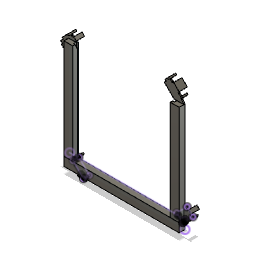
ClipOn v35 (Autodesk Fusion 360 design; units mm, degrees)
Autodesk Fusion 360 part; units mm, degrees
(part 1 of 2)
sketch "Sketch1" plane through (0, 0, 0) normal (0, 0, 1) x (1, 0, 0) in component "Faceplate"
  line L0 (10, 10) -> (310, 10)
  line L1 (310, 10) -> (310, 360)
  line L2 (310, 360) -> (10, 360)
  line L3 (10, 360) -> (10, 10)
  line L4 (85, 300) -> (235, 300)
  line L5 (235, 300) -> (235, 150)
  line L6 (235, 150) -> (85, 150)
  line L7 (85, 150) -> (85, 300)
  dimension "d7" = 10
  dimension "d8" = 10
  dimension "d10" = 350
  dimension "d11" = 75
  dimension "d12" = 140
  dimension "d13" = 150
  dimension "d14" = 150
  dimension "d15" = 75
  constraint horizontal L0
  constraint vertical L1
  constraint horizontal L2
  constraint vertical L3
  constraint horizontal L4
  constraint vertical L5
  constraint horizontal L6
  constraint vertical L7
  measures "d7" horizontal distance of origin L0.start
  measures "d8" vertical distance of origin L0.start
  measures "d10" distance of L0.end L1.end
  measures "d11" horizontal distance of L0.start L6.end
  measures "d12" vertical distance of L0.start L6.end
  measures "d13" distance of L5.end L6.end
  measures "d14" distance of L4.end L5.end
  measures "d15" horizontal distance of L0.end L5.end
extrude "Extrude1" add sketch "Sketch1" against normal blind 10 makes body 1 in component "Faceplate"
sketch "Sketch2" plane through (0, 0, 0) normal (0, 0, 1) x (1, 0, 0) in component "Bottom holder OLD"
  line L0 (235, 150) -> (85, 150)
  line L1 (85, 150) -> (85, 300)
  line L2 (85, 300) -> (235, 300)
  line L3 (235, 300) -> (235, 150)
  line L4 (10, 360) -> (10, 10)
  line L5 (10, 10) -> (310, 10)
  line L6 (310, 10) -> (310, 360)
  line L7 (310, 360) -> (10, 360)
  line L8 (258, 125) -> (62, 125)
  line L9 (62, 125) -> (62, 140)
  line L10 (62, 140) -> (258, 140)
  line L11 (258, 125) -> (258, 140)
  dimension "d18" = 196
  dimension "d20" = 15
  dimension "d69" = 10
  dimension "d70" = 23
  dimension "d74" = 15
  constraint horizontal L8
  constraint vertical L9
  constraint perpendicular L9 L10
  constraint perpendicular L10 L11
  measures "d18" distance of L8.start L8.end
  measures "d20" distance of L9.end L8.end
  measures "d69" vertical distance of L0.start L10.end
  measures "d70" horizontal distance of L0.end L9.end
  measures "d74" distance of L8.start L10.end
sketch "Sketch1 (2)" plane through (0, 0, 0) normal (0, 0, 1) x (1, 0, 0) in component "Left holder OLD"
  line L0 (235, 150) -> (85, 150)
  line L1 (85, 150) -> (85, 300)
  line L2 (85, 300) -> (235, 300)
  line L3 (235, 300) -> (235, 150)
  line L4 (10, 360) -> (10, 10)
  line L5 (10, 10) -> (310, 10)
  line L6 (310, 10) -> (310, 360)
  line L7 (310, 360) -> (10, 360)
  line L8 (77, 310) -> (62, 310)
  line L9 (62, 310) -> (62, 140)
  line L10 (62, 140) -> (77, 140)
  line L11 (77, 140) -> (77, 310)
  dimension "d23" = 15
  dimension "d24" = 170
  dimension "d64" = 10
  dimension "d72" = 8
  constraint horizontal L8
  constraint vertical L9
  constraint horizontal L10
  constraint vertical L11
  measures "d23" distance of L8.start L8.end
  measures "d24" distance of L8.end L9.end
  measures "d64" vertical distance of L0.end L10.end
  measures "d72" horizontal distance of L1.end L8.start
sketch "Sketch1 (3)" plane through (0, 0, 0) normal (0, 0, 1) x (1, 0, 0) in component "Right holder OLD"
  line L0 (235, 150) -> (85, 150)
  line L1 (85, 150) -> (85, 300)
  line L2 (85, 300) -> (241.0837, 300)
  line L3 (235, 300) -> (235, 150)
  line L4 (10, 360) -> (10, 10)
  line L5 (10, 10) -> (310, 10)
  line L6 (310, 10) -> (310, 360)
  line L7 (310, 360) -> (10, 360)
  line L8 (258, 310) -> (258, 140)
  line L9 (243, 140) -> (243, 310)
  line L10 (243, 140) -> (258, 140)
  line L11 (258, 310) -> (243, 310)
  dimension "d21" = 15
  dimension "d66" = 10
  dimension "d67" = 170
  dimension "d73" = 8
  constraint vertical L8
  constraint vertical L9
  constraint perpendicular L8 L10
  constraint perpendicular L9 L11
  measures "d21" distance of L9.end L8.start
  measures "d66" vertical distance of L0.start L9.start
  measures "d67" distance of L8.start L8.end
  measures "d73" horizontal distance of L3.start L9.end
extrude "Extrude2" add sketch "Sketch2" along normal blind 10 separate body contours L8 L9 L10 L11 makes body 2 in component "Bottom holder OLD"
extrude "Extrude1'" add sketch "Sketch1 (2)" along normal blind 10 separate body contours L8 L9 L10 L11 makes body 3 in component "Left holder OLD"
extrude "Extrude1''" add sketch "Sketch1 (3)" along normal blind 10 separate body contours L8 L9 L10 L11 makes body 4 in component "Right holder OLD"
sketch "Sketch2 (2)" plane through (77, 0, 0) normal (1, 0, 0) x (0, 0, -1) in component "Left holder OLD"
  line L0 (0, 140) -> (0, 310)
  line L1 (0, 310) -> (-10, 310)
  line L2 (-10, 310) -> (-10, 140)
  line L3 (-10, 140) -> (0, 140)
  line L4 (0, 310) -> (-1.5, 310)
  line L5 (-1.5, 310) -> (-1.5, 140)
  line L6 (-1.5, 140) -> (0, 140)
  line L7 (0, 140) -> (0, 310)
  dimension "d31" = 1.5
  constraint horizontal L4
  constraint vertical L5
  constraint horizontal L6
  constraint vertical L7
  constraint coincident L3 L5.end
  constraint coincident L0.end L1.start
  measures "d31" distance of L0.end L4.end
extrude "Extrude2'" cut sketch "Sketch2 (2)" against normal blind 3 contours L0 L1 L3 L4 L5 L6 L7 bodies 3 in component "Left holder OLD"
sketch "Sketch2 (3)" plane through (243, 0, 0) normal (-1, 0, 0) x (0, 0, 1) in component "Right holder OLD"
  line L0 (0, 310) -> (0, 140)
  line L1 (10, 140) -> (10, 310)
  line L2 (0, 310) -> (1.5, 310)
  line L3 (1.5, 310) -> (1.5, 145)
  line L4 (1.5, 145) -> (0, 145)
  line L5 (0, 145) -> (0, 310)
  line L6 (0, 140) -> (10, 140)
  line L7 (10, 310) -> (0, 310)
  dimension "d34" = 1.5
  constraint horizontal L2
  constraint vertical L3
  constraint horizontal L4
  constraint vertical L5
  constraint coincident L0.start L2.start
  measures "d34" distance of L3.end L4.end
extrude "Extrude2''" cut sketch "Sketch2 (3)" against normal blind 3 contours L0 L2 L3 L4 L5 L7 bodies 4 in component "Right holder OLD"
sketch "Sketch3" plane through (0, 0, 0) normal (0, 0, -1) x (-1, 0, 0) in component "Bottom holder OLD"
  line L0 (-258, 125) -> (-62, 125)
  line L1 (-62, 125) -> (-62, 140)
  circle A0 centre (-218, 132.5) radius 2.25
  circle A1 centre (-102, 132.5) radius 2.25
  line L2 (-62, 140) -> (-258, 140)
  line L3 (-258, 140) -> (-258, 125)
  dimension "d37" = 40
  dimension "d38" = 7.5
  dimension "d39" = 40
  dimension "d40" = 7.5
  dimension "d41" = 4.5
  dimension "d42" = 4.5
  measures "d37" horizontal distance of L0.start A0.centre
  measures "d38" vertical distance of L0.start A0.centre
  measures "d39" horizontal distance of L0.end A1.centre
  measures "d40" vertical distance of L0.end A1.centre
  measures "d41" diameter of A1
  measures "d42" diameter of A0
extrude "Extrude3" cut sketch "Sketch3" against normal blind 7 contours A0 | A1 bodies 2 in component "Bottom holder OLD"
sketch "Sketch3 (2)" plane through (0, 0, 0) normal (0, 0, -1) x (-1, 0, 0) in component "Left holder OLD"
  line L0 (-74, 310) -> (-74, 140)
  line L1 (-74, 140) -> (-62, 140)
  line L2 (-62, 140) -> (-62, 310)
  line L3 (-62, 310) -> (-74, 310)
  circle A0 centre (-68.5, 290) radius 2.25
  circle A1 centre (-68.5, 160) radius 2.25
  dimension "d45" = 20
  dimension "d46" = 20
  dimension "d47" = 6.5
  dimension "d48" = 6.5
  dimension "d49" = 4.5
  dimension "d50" = 4.5
  measures "d45" vertical distance of L2.end A0.centre
  measures "d46" vertical distance of L1.end A1.centre
  measures "d47" horizontal distance of L2.end A0.centre
  measures "d48" horizontal distance of L1.end A1.centre
  measures "d49" diameter of A0
  measures "d50" diameter of A1
sketch "Sketch3 (3)" plane through (0, 0, 0) normal (0, 0, -1) x (-1, 0, 0) in component "Right holder OLD"
  line L0 (-246, 145) -> (-246, 310)
  line L1 (-258, 310) -> (-258, 140)
  circle A0 centre (-251.5, 290) radius 2.25
  circle A1 centre (-251.5, 160) radius 2.25
  line L2 (-246, 310) -> (-258, 310)
  line L3 (-258, 140) -> (-243, 140)
  line L4 (-243, 140) -> (-243, 145)
  line L5 (-243, 145) -> (-246, 145)
  dimension "d52" = 20
  dimension "d53" = 20
  dimension "d55" = 6.5
  dimension "d56" = 6.5
  dimension "d57" = 4.5
  dimension "d58" = 4.5
  measures "d52" vertical distance of L1.start A0.centre
  measures "d53" vertical distance of L1.end A1.centre
  measures "d55" horizontal distance of L1.start A0.centre
  measures "d56" horizontal distance of L1.end A1.centre
  measures "d57" diameter of A1
  measures "d58" diameter of A0
extrude "Extrude3'" cut sketch "Sketch3 (2)" against normal blind 7 contours A0 | A1 bodies 3 in component "Left holder OLD"
extrude "Extrude3''" cut sketch "Sketch3 (3)" against normal blind 7 contours A0 | A1 bodies 4 in component "Right holder OLD"
ref_plane "WorkPlane1" through (160, 185, -60) normal (0, 0, -1) x (-1, 0, 0) in component "Bottom holder OLD"
sketch "Sketch1 (4)" plane through (160, 185, -60) normal (0, 0, -1) x (1, 0, 0) in component "Backplate"
  line L0 (150, -175) -> (-150, -175)
  line L1 (-150, -175) -> (-150, 175)
  line L2 (-150, 175) -> (150, 175)
  line L3 (150, 175) -> (150, -175)
  line L4 (75, -115) -> (-75, -115)
  line L5 (-75, -115) -> (-75, 35)
  line L6 (-75, 35) -> (75, 35)
  line L7 (75, 35) -> (75, -115)
  dimension "d76" = 300
  dimension "d77" = 350
  dimension "d78" = 175
  dimension "d79" = 150
  dimension "d84" = 150
  dimension "d85" = 150
  dimension "d86" = 75
  dimension "d87" = 60
  constraint horizontal L0
  constraint vertical L1
  constraint horizontal L2
  constraint vertical L3
  constraint horizontal L4
  constraint vertical L5
  constraint horizontal L6
  constraint vertical L7
  measures "d76" distance of L1.end L2.end
  measures "d77" distance of L0.start L2.end
  measures "d78" vertical distance of origin L1.end
  measures "d79" horizontal distance of origin L1.end
  measures "d84" distance of L4.start L6.end
  measures "d85" distance of L4.start L4.end
  measures "d86" distance of L3 L6.end
  measures "d87" distance of L0 L4.start
extrude "Extrude1'''" add sketch "Sketch1 (4)" along normal blind 20 separate body makes body 5 in component "Backplate"
sketch "Sketch1 (5)" plane through (0, 0, -60) normal (0, 0, 1) x (1, 0, 0) in component "Help lines"
  line L0 (235, 150) -> (85, 150)
  line L1 (85, 150) -> (85, 300)
  line L2 (85, 300) -> (235, 300)
  line L3 (235, 300) -> (235, 150)
  line L4 (10, 10) -> (310, 10)
  line L5 (310, 10) -> (310, 360)
  line L6 (310, 360) -> (10, 360)
  line L7 (10, 360) -> (10, 10)
  line L8 (85, 300) -> (235, 150)
  line L9 (85, 150) -> (235, 300)
  circle A0 centre (160, 225) radius 115
  line L10 (160, 225) -> (78.6827, 143.6827)
  line L11 (160, 225) -> (241.3173, 143.6827)
  line L12 (160, 225) -> (241.3173, 306.3173)
  line L13 (160, 225) -> (78.6827, 306.3173)
  circle A1 centre (160, 225) radius 118
  line L14 (160, 225) -> (76.5614, 141.5614)
  line L15 (160, 225) -> (243.4386, 141.5614)
  line L16 (160, 225) -> (243.4386, 308.4386)
  line L17 (160, 225) -> (76.5614, 308.4386)
  dimension "d90" = 230
  dimension "d131" = 236
  constraint coincident L1.end L2.start
  constraint coincident L0.start L3.end
  constraint coincident L0.end L1.start
  constraint coincident L2.end L3.start
  constraint midpoint L8 A0.centre
  constraint coincident A0.centre L10.start
  constraint coincident A0 L10.end
  constraint parallel L9 L10
  constraint coincident A0 L11.end
  constraint perpendicular L10 L11
  constraint coincident A0 L12.end
  constraint perpendicular L11 L12
  constraint coincident A0 L13.end
  constraint perpendicular L12 L13
  constraint concentric A0 A1
  constraint coincident A1 L14.end
  constraint parallel L9 L14
  constraint coincident A1 L15.end
  constraint perpendicular L14 L15
  constraint coincident A1 L16.end
  constraint perpendicular L15 L16
  constraint coincident A1 L17.end
  constraint perpendicular L16 L17
  measures "d90" diameter of A0
  measures "d131" diameter of A1
sketch "Sketch2 (4)" plane through (0, 0, -60) normal (0, 0, 1) x (1, 0, 0) in component "Sensor-Holder West"
  line L0 (235, 150) -> (85, 150)
  line L1 (85, 150) -> (85, 300)
  line L2 (85, 300) -> (235, 300)
  line L3 (235, 300) -> (235, 150)
  line L4 (10, 10) -> (310, 10)
  line L5 (310, 10) -> (310, 360)
  line L6 (310, 360) -> (10, 360)
  line L7 (10, 360) -> (10, 10)
  line L8 (78.8806, 143.4853) -> (96.5583, 125.8076)
  line L9 (96.5583, 125.8076) -> (88.073, 117.3223)
  line L10 (88.073, 117.3223) -> (70.3954, 135)
  line L11 (70.3954, 135) -> (78.8806, 143.4853)
  circle A0 centre (160, 225) radius 115
  point P0 (85, 150)
  dimension "d91" = 12
  dimension "d92" = 25
  dimension "d93" = 15
  dimension "d94" = 45
  constraint perpendicular L8 L9
  constraint parallel L8 L10
  constraint parallel L9 L11
  constraint coincident L8.start A0
  measures "d91" distance of L8.start L10.end
  measures "d92" distance of L9.end L10.end
  measures "d93" vertical distance of L10.end P0
  measures "d94" angle of L7 L10
extrude "Extrude1''''" add sketch "Sketch2 (4)" along normal blind 24.5 separate body contours L8 L9 L10 L11 makes body 6 in component "Sensor-Holder West"
sketch "Sketch3 (4)" plane through (111.183, 111.183, 0) normal (0.707107, 0.707107, 0) x (0, 0, -1) in component "Sensor-Holder West"
  line L0 (60, 20.6824) -> (60, 45.6824)
  line L1 (60, 45.6824) -> (35.5, 45.6824)
  line L2 (35.5, 45.6824) -> (35.5, 20.6824)
  line L3 (35.5, 20.6824) -> (60, 20.6824)
  line L4 (60, 45.6824) -> (59, 45.6824)
  line L5 (59, 45.6824) -> (59, 20.6824)
  line L6 (59, 20.6824) -> (60, 20.6824)
  line L7 (60, 20.6824) -> (60, 45.6824)
  point P0 (60, 45.9619)
  dimension "d97" = 1
  constraint horizontal L4
  constraint vertical L5
  constraint horizontal L6
  constraint vertical L7
  constraint coincident L3 L5.end
  constraint coincident L0.end L1.start
  measures "d97" horizontal distance of L4.end P0
extrude "Extrude2'''" add sketch "Sketch3 (4)" along normal blind 2 contours L0 L1 L3 L4 L5 L6 L7 bodies 6 in component "Sensor-Holder West"
sketch "Sketch4" plane through (111.183, 111.183, 0) normal (0.707107, 0.707107, 0) x (0, 0, -1) in component "Sensor-Holder West"
  line L0 (59, 20.6824) -> (59, 45.6824)
  line L1 (59, 45.6824) -> (35.5, 45.6824)
  line L2 (35.5, 45.6824) -> (35.5, 20.6824)
  line L3 (35.5, 20.6824) -> (59, 20.6824)
  circle A0 centre (38.5, 38.6824) radius 1.5
  circle A1 centre (38.5, 24.6824) radius 1.5
  dimension "d100" = 3
  dimension "d101" = 3
  dimension "d102" = 14
  dimension "d103" = 20.5
  dimension "d104" = 7
  dimension "d105" = 20.5
  measures "d100" diameter of A0
  measures "d101" diameter of A1
  measures "d102" distance of A0.centre A1.centre
  measures "d103" horizontal distance of L0.end A0.centre
  measures "d104" vertical distance of L1.end A0.centre
  measures "d105" horizontal distance of L0.start A1.centre
extrude "Extrude3'''" add sketch "Sketch4" along normal blind 3 contours A0 bodies 6 in component "Sensor-Holder West"
extrude "Extrude4" add sketch "Sketch4" along normal up to surface (3 mm away) contours A1 bodies 6 in component "Sensor-Holder West"
sketch "Sketch1 (6)" plane through (0, 0, -35.4282) normal (0, 0, -1) x (-1, 0, 0)
  line L0 (-62, 310) -> (-77, 310)
  line L1 (-77, 310) -> (-77, 140)
  line L2 (-77, 140) -> (-62, 140)
  line L3 (-62, 140) -> (-62, 310)
sketch "Sketch1 (7)" plane through (111.183, 111.183, 0) normal (0.707107, 0.707107, 0) x (0, 0, -1) in component "Sensor West"
  circle A0 centre (38.5, 24.6824) radius 1.5
  circle A1 centre (38.5, 38.6824) radius 1.5
  line L0 (59, 20.6824) -> (59, 45.6824)
  line L1 (59, 45.6824) -> (35.5, 45.6824)
  line L2 (35.5, 45.6824) -> (35.5, 20.6824)
  line L3 (35.5, 20.6824) -> (59, 20.6824)
  line L4 (59, 53.6824) -> (36, 53.6824)
  line L5 (36, 53.6824) -> (36, 7.6824)
  line L6 (36, 7.6824) -> (59, 7.6824)
  line L7 (59, 7.6824) -> (59, 53.6824)
  line L8 (60, 35.3553) -> (60, 247.4874)
  dimension "d111" = 8
  dimension "d113" = 46
  dimension "d114" = 23
  dimension "d115" = 1
  constraint horizontal L4
  constraint vertical L5
  constraint horizontal L6
  constraint vertical L7
  measures "d111" vertical distance of L1.end L4.end
  measures "d113" distance of L4.end L5.end
  measures "d114" distance of L5.end L6.end
  measures "d115" distance of L4.start L8
extrude "Extrude1'''''" add sketch "Sketch1 (7)" along normal blind 1.6 separate body contours L0 L1 L3 L5 L7 | L3 L5 L6 L7 | L1 L4 L5 L7 makes body 8 in component "Sensor West"
sketch "Sketch2 (5)" plane through (112.3143, 112.3143, 0) normal (0.707107, 0.707107, 0) x (0, 0, -1) in component "Sensor West"
  circle A0 centre (38.5, 24.6824) radius 1.5
  circle A1 centre (38.5, 38.6824) radius 1.5
  line L0 (59, 7.6824) -> (59, 53.6824)
  line L1 (59, 53.6824) -> (36, 53.6824)
  line L2 (36, 53.6824) -> (36, 7.6824)
  line L3 (36, 7.6824) -> (59, 7.6824)
  circle A2 centre (44, 46.6824) radius 3
  line L4 (37.0281, 7.6824) -> (56, 7.6824)
  line L5 (36, 7.6824) -> (59, 7.6824)
  line L6 (59, 7.6824) -> (59, 16.3824)
  line L7 (59, 16.3824) -> (36, 16.3824)
  line L8 (36, 16.3824) -> (36, 7.6824)
  line L9 (44, 46.6824) -> (59, 46.6824)
  dimension "d119" = 7
  dimension "d124" = 6
  dimension "d125" = 8
  dimension "d126" = 8.7
  constraint horizontal L4
  constraint coincident L3 L4.start
  constraint horizontal L5
  constraint vertical L6
  constraint horizontal L7
  constraint vertical L8
  constraint coincident L0 L6.end
  constraint coincident L2.end L3.start
  constraint coincident A2.centre L9.start
  constraint coincident L0 L9.end
  constraint perpendicular L0 L9
  measures "d119" vertical distance of L1.end A2.centre
  measures "d124" diameter of A2
  measures "d125" horizontal distance of L1.end A2.centre
  measures "d126" distance of L2.end L7.end
extrude "Extrude2''''" add sketch "Sketch2 (5)" along normal blind 3 contours A2 bodies 8 in component "Sensor West"
extrude "Extrude4'" add sketch "Sketch2 (5)" along normal blind 8.9 contours L0 L2 L3 L4 L5 L6 L7 L8 bodies 8 in component "Sensor West"
extrude "Extrude3''''" add sketch "Sketch1 (5)" along normal blind 1 separate body contours A0 A1 L14 L15 | A0 A1 L15 L16 | A0 A1 L14 L17 | A0 A1 L16 L17 makes body 9 in component "Help lines"
sketch "Sketch2 (6)" plane through (0, 0, -60) normal (0, 0, 1) x (1, 0, 0) in component "Sensor-Holder South"
  line L0 (235, 150) -> (85, 150)
  line L1 (85, 150) -> (85, 300)
  line L2 (85, 300) -> (235, 300)
  line L3 (235, 300) -> (235, 150)
  line L4 (10, 10) -> (310, 10)
  line L5 (310, 10) -> (310, 360)
  line L6 (310, 360) -> (10, 360)
  line L7 (10, 360) -> (10, 10)
  line L8 (78.8806, 143.4853) -> (96.5583, 125.8076)
  line L9 (96.5583, 125.8076) -> (88.073, 117.3223)
  line L10 (88.073, 117.3223) -> (70.3954, 135)
  line L11 (70.3954, 135) -> (78.8806, 143.4853)
  circle A0 centre (160, 225) radius 115
  point P0 (85, 150)
  dimension "d91_1" = 12
  dimension "d92_1" = 25
  dimension "d93_1" = 15
  dimension "d94_1" = 45
  constraint perpendicular L8 L9
  constraint parallel L8 L10
  constraint parallel L9 L11
  constraint coincident L8.start A0
  measures "d91_1" distance of L8.start L10.end
  measures "d92_1" distance of L9.end L10.end
  measures "d93_1" vertical distance of L10.end P0
  measures "d94_1" angle of L7 L10
extrude "Extrude1''''''" add sketch "Sketch2 (6)" along normal blind 24.5 separate body contours L8 L9 L10 L11 makes body 10 in component "Sensor-Holder South"
sketch "Sketch3 (5)" plane through (111.183, 111.183, 0) normal (0.707107, 0.707107, 0) x (0, 0, -1) in component "Sensor-Holder South"
  line L0 (60, 20.6824) -> (60, 45.6824)
  line L1 (60, 45.6824) -> (35.5, 45.6824)
  line L2 (35.5, 45.6824) -> (35.5, 20.6824)
  line L3 (35.5, 20.6824) -> (60, 20.6824)
  line L4 (60, 45.6824) -> (59, 45.6824)
  line L5 (59, 45.6824) -> (59, 20.6824)
  line L6 (59, 20.6824) -> (60, 20.6824)
  line L7 (60, 20.6824) -> (60, 45.6824)
  point P0 (60, 45.9619)
  dimension "d97_1" = 1
  constraint horizontal L4
  constraint vertical L5
  constraint horizontal L6
  constraint vertical L7
  constraint coincident L3 L5.end
  constraint coincident L0.end L1.start
  measures "d97_1" horizontal distance of L4.end P0
extrude "Extrude2'''''" add sketch "Sketch3 (5)" along normal blind 2 contours L0 L1 L3 L4 L5 L6 L7 bodies 10 in component "Sensor-Holder South"
sketch "Sketch4 (2)" plane through (111.183, 111.183, 0) normal (0.707107, 0.707107, 0) x (0, 0, -1) in component "Sensor-Holder South"
  line L0 (59, 20.6824) -> (59, 45.6824)
  line L1 (59, 45.6824) -> (35.5, 45.6824)
  line L2 (35.5, 45.6824) -> (35.5, 20.6824)
  line L3 (35.5, 20.6824) -> (59, 20.6824)
  circle A0 centre (38.5, 38.6824) radius 1.5
  circle A1 centre (38.5, 24.6824) radius 1.5
  dimension "d100_1" = 3
  dimension "d101_1" = 3
  dimension "d102_1" = 14
  dimension "d103_1" = 20.5
  dimension "d104_1" = 7
  dimension "d105_1" = 20.5
  measures "d100_1" diameter of A0
  measures "d101_1" diameter of A1
  measures "d102_1" distance of A0.centre A1.centre
  measures "d103_1" horizontal distance of L0.end A0.centre
  measures "d104_1" vertical distance of L1.end A0.centre
  measures "d105_1" horizontal distance of L0.start A1.centre
extrude "Extrude3'''''" add sketch "Sketch4 (2)" along normal blind 3 contours A0 bodies 10 in component "Sensor-Holder South"
extrude "Extrude4''" add sketch "Sketch4 (2)" along normal up to surface (3 mm away) contours A1 bodies 10 in component "Sensor-Holder South"
sketch "Sketch1 (8)" plane through (111.183, 111.183, 0) normal (0.707107, 0.707107, 0) x (0, 0, -1) in component "Sensor South"
  circle A0 centre (38.5, 24.6824) radius 1.5
  circle A1 centre (38.5, 38.6824) radius 1.5
  line L0 (59, 20.6824) -> (59, 45.6824)
  line L1 (59, 45.6824) -> (35.5, 45.6824)
  line L2 (35.5, 45.6824) -> (35.5, 20.6824)
  line L3 (35.5, 20.6824) -> (59, 20.6824)
  line L4 (59, 53.6824) -> (36, 53.6824)
  line L5 (36, 53.6824) -> (36, 7.6824)
  line L6 (36, 7.6824) -> (59, 7.6824)
  line L7 (59, 7.6824) -> (59, 53.6824)
  line L8 (60, 35.3553) -> (60, 247.4874)
  dimension "d111_1" = 8
  dimension "d113_1" = 46
  dimension "d114_1" = 23
  dimension "d115_1" = 1
  constraint horizontal L4
  constraint vertical L5
  constraint horizontal L6
  constraint vertical L7
  measures "d111_1" vertical distance of L1.end L4.end
  measures "d113_1" distance of L4.end L5.end
  measures "d114_1" distance of L5.end L6.end
  measures "d115_1" distance of L4.start L8
extrude "Extrude1'''''''" add sketch "Sketch1 (8)" along normal blind 1.6 separate body contours L0 L1 L3 L5 L7 | L3 L5 L6 L7 | L1 L4 L5 L7 makes body 11 in component "Sensor South"
sketch "Sketch2 (7)" plane through (112.3143, 112.3143, 0) normal (0.707107, 0.707107, 0) x (0, 0, -1) in component "Sensor South"
  circle A0 centre (38.5, 24.6824) radius 1.5
  circle A1 centre (38.5, 38.6824) radius 1.5
  line L0 (59, 7.6824) -> (59, 53.6824)
  line L1 (59, 53.6824) -> (36, 53.6824)
  line L2 (36, 53.6824) -> (36, 7.6824)
  line L3 (36, 7.6824) -> (59, 7.6824)
  circle A2 centre (44, 46.6824) radius 3
  line L4 (37.0281, 7.6824) -> (56, 7.6824)
  line L5 (36, 7.6824) -> (59, 7.6824)
  line L6 (59, 7.6824) -> (59, 16.3824)
  line L7 (59, 16.3824) -> (36, 16.3824)
  line L8 (36, 16.3824) -> (36, 7.6824)
  line L9 (44, 46.6824) -> (59, 46.6824)
  dimension "d119_1" = 7
  dimension "d124_1" = 6
  dimension "d125_1" = 8
  dimension "d126_1" = 8.7
  constraint horizontal L4
  constraint coincident L3 L4.start
  constraint horizontal L5
  constraint vertical L6
  constraint horizontal L7
  constraint vertical L8
  constraint coincident L0 L6.end
  constraint coincident L2.end L3.start
  constraint coincident A2.centre L9.start
  constraint coincident L0 L9.end
  constraint perpendicular L0 L9
  measures "d119_1" vertical distance of L1.end A2.centre
  measures "d124_1" diameter of A2
  measures "d125_1" horizontal distance of L1.end A2.centre
  measures "d126_1" distance of L2.end L7.end
extrude "Extrude2''''''" add sketch "Sketch2 (7)" along normal blind 3 contours A2 bodies 11 in component "Sensor South"
extrude "Extrude4'''" add sketch "Sketch2 (7)" along normal blind 8.9 contours L0 L2 L3 L4 L5 L6 L7 L8 bodies 11 in component "Sensor South"
sketch "Sketch2 (8)" plane through (0, 0, -60) normal (0, 0, 1) x (1, 0, 0) in component "Sensor-Holder North"
  line L0 (235, 150) -> (85, 150)
  line L1 (85, 150) -> (85, 300)
  line L2 (85, 300) -> (235, 300)
  line L3 (235, 300) -> (235, 150)
  line L4 (10, 10) -> (310, 10)
  line L5 (310, 10) -> (310, 360)
  line L6 (310, 360) -> (10, 360)
  line L7 (10, 360) -> (10, 10)
  line L8 (78.8806, 143.4853) -> (96.5583, 125.8076)
  line L9 (96.5583, 125.8076) -> (88.073, 117.3223)
  line L10 (88.073, 117.3223) -> (70.3954, 135)
  line L11 (70.3954, 135) -> (78.8806, 143.4853)
  circle A0 centre (160, 225) radius 115
  point P0 (85, 150)
  dimension "d91_2" = 12
  dimension "d92_2" = 25
  dimension "d93_2" = 15
  dimension "d94_2" = 45
  constraint perpendicular L8 L9
  constraint parallel L8 L10
  constraint parallel L9 L11
  constraint coincident L8.start A0
  measures "d91_2" distance of L8.start L10.end
  measures "d92_2" distance of L9.end L10.end
  measures "d93_2" vertical distance of L10.end P0
  measures "d94_2" angle of L7 L10
extrude "Extrude1''''''''" add sketch "Sketch2 (8)" along normal blind 24.5 separate body contours L8 L9 L10 L11 makes body 12 in component "Sensor-Holder North"
sketch "Sketch3 (6)" plane through (111.183, 111.183, 0) normal (0.707107, 0.707107, 0) x (0, 0, -1) in component "Sensor-Holder North"
  line L0 (60, 20.6824) -> (60, 45.6824)
  line L1 (60, 45.6824) -> (35.5, 45.6824)
  line L2 (35.5, 45.6824) -> (35.5, 20.6824)
  line L3 (35.5, 20.6824) -> (60, 20.6824)
  line L4 (60, 45.6824) -> (59, 45.6824)
  line L5 (59, 45.6824) -> (59, 20.6824)
  line L6 (59, 20.6824) -> (60, 20.6824)
  line L7 (60, 20.6824) -> (60, 45.6824)
  point P0 (60, 45.9619)
  dimension "d97_2" = 1
  constraint horizontal L4
  constraint vertical L5
  constraint horizontal L6
  constraint vertical L7
  constraint coincident L3 L5.end
  constraint coincident L0.end L1.start
  measures "d97_2" horizontal distance of L4.end P0
extrude "Extrude2'''''''" add sketch "Sketch3 (6)" along normal blind 2 contours L0 L1 L3 L4 L5 L6 L7 bodies 12 in component "Sensor-Holder North"
sketch "Sketch4 (3)" plane through (111.183, 111.183, 0) normal (0.707107, 0.707107, 0) x (0, 0, -1) in component "Sensor-Holder North"
  line L0 (59, 20.6824) -> (59, 45.6824)
  line L1 (59, 45.6824) -> (35.5, 45.6824)
  line L2 (35.5, 45.6824) -> (35.5, 20.6824)
  line L3 (35.5, 20.6824) -> (59, 20.6824)
  circle A0 centre (38.5, 38.6824) radius 1.5
  circle A1 centre (38.5, 24.6824) radius 1.5
  dimension "d100_2" = 3
  dimension "d101_2" = 3
  dimension "d102_2" = 14
  dimension "d103_2" = 20.5
  dimension "d104_2" = 7
  dimension "d105_2" = 20.5
  measures "d100_2" diameter of A0
  measures "d101_2" diameter of A1
  measures "d102_2" distance of A0.centre A1.centre
  measures "d103_2" horizontal distance of L0.end A0.centre
  measures "d104_2" vertical distance of L1.end A0.centre
  measures "d105_2" horizontal distance of L0.start A1.centre
extrude "Extrude3''''''" add sketch "Sketch4 (3)" along normal blind 3 contours A0 bodies 12 in component "Sensor-Holder North"
extrude "Extrude4''''" add sketch "Sketch4 (3)" along normal up to surface (3 mm away) contours A1 bodies 12 in component "Sensor-Holder North"
sketch "Sketch1 (9)" plane through (111.183, 111.183, 0) normal (0.707107, 0.707107, 0) x (0, 0, -1) in component "Sensor North"
  circle A0 centre (38.5, 24.6824) radius 1.5
  circle A1 centre (38.5, 38.6824) radius 1.5
  line L0 (59, 20.6824) -> (59, 45.6824)
  line L1 (59, 45.6824) -> (35.5, 45.6824)
  line L2 (35.5, 45.6824) -> (35.5, 20.6824)
  line L3 (35.5, 20.6824) -> (59, 20.6824)
  line L4 (59, 53.6824) -> (36, 53.6824)
  line L5 (36, 53.6824) -> (36, 7.6824)
  line L6 (36, 7.6824) -> (59, 7.6824)
  line L7 (59, 7.6824) -> (59, 53.6824)
  line L8 (60, 35.3553) -> (60, 247.4874)
  dimension "d111_2" = 8
  dimension "d113_2" = 46
  dimension "d114_2" = 23
  dimension "d115_2" = 1
  constraint horizontal L4
  constraint vertical L5
  constraint horizontal L6
  constraint vertical L7
  measures "d111_2" vertical distance of L1.end L4.end
  measures "d113_2" distance of L4.end L5.end
  measures "d114_2" distance of L5.end L6.end
  measures "d115_2" distance of L4.start L8
extrude "Extrude1'''''''''" add sketch "Sketch1 (9)" along normal blind 1.6 separate body contours L0 L1 L3 L5 L7 | L3 L5 L6 L7 | L1 L4 L5 L7 makes body 13 in component "Sensor North"
sketch "Sketch2 (9)" plane through (112.3143, 112.3143, 0) normal (0.707107, 0.707107, 0) x (0, 0, -1) in component "Sensor North"
  circle A0 centre (38.5, 24.6824) radius 1.5
  circle A1 centre (38.5, 38.6824) radius 1.5
  line L0 (59, 7.6824) -> (59, 53.6824)
  line L1 (59, 53.6824) -> (36, 53.6824)
  line L2 (36, 53.6824) -> (36, 7.6824)
  line L3 (36, 7.6824) -> (59, 7.6824)
  circle A2 centre (44, 46.6824) radius 3
  line L4 (37.0281, 7.6824) -> (56, 7.6824)
  line L5 (36, 7.6824) -> (59, 7.6824)
  line L6 (59, 7.6824) -> (59, 16.3824)
  line L7 (59, 16.3824) -> (36, 16.3824)
  line L8 (36, 16.3824) -> (36, 7.6824)
  line L9 (44, 46.6824) -> (59, 46.6824)
  dimension "d119_2" = 7
  dimension "d124_2" = 6
  dimension "d125_2" = 8
  dimension "d126_2" = 8.7
  constraint horizontal L4
  constraint coincident L3 L4.start
  constraint horizontal L5
  constraint vertical L6
  constraint horizontal L7
  constraint vertical L8
  constraint coincident L0 L6.end
  constraint coincident L2.end L3.start
  constraint coincident A2.centre L9.start
  constraint coincident L0 L9.end
  constraint perpendicular L0 L9
  measures "d119_2" vertical distance of L1.end A2.centre
  measures "d124_2" diameter of A2
  measures "d125_2" horizontal distance of L1.end A2.centre
  measures "d126_2" distance of L2.end L7.end
extrude "Extrude2''''''''" add sketch "Sketch2 (9)" along normal blind 3 contours A2 bodies 13 in component "Sensor North"
extrude "Extrude4'''''" add sketch "Sketch2 (9)" along normal blind 8.9 contours L0 L2 L3 L4 L5 L6 L7 L8 bodies 13 in component "Sensor North"
sketch "Sketch2 (10)" plane through (0, 0, -60) normal (0, 0, 1) x (1, 0, 0) in component "Sensor-Holder East"
  line L0 (235, 150) -> (85, 150)
  line L1 (85, 150) -> (85, 300)
  line L2 (85, 300) -> (235, 300)
  line L3 (235, 300) -> (235, 150)
  line L4 (10, 10) -> (310, 10)
  line L5 (310, 10) -> (310, 360)
  line L6 (310, 360) -> (10, 360)
  line L7 (10, 360) -> (10, 10)
  line L8 (78.8806, 143.4853) -> (96.5583, 125.8076)
  line L9 (96.5583, 125.8076) -> (88.073, 117.3223)
  line L10 (88.073, 117.3223) -> (70.3954, 135)
  line L11 (70.3954, 135) -> (78.8806, 143.4853)
  circle A0 centre (160, 225) radius 115
  point P0 (85, 150)
  dimension "d91_3" = 12
  dimension "d92_3" = 25
  dimension "d93_3" = 15
  dimension "d94_3" = 45
  constraint perpendicular L8 L9
  constraint parallel L8 L10
  constraint parallel L9 L11
  constraint coincident L8.start A0
  measures "d91_3" distance of L8.start L10.end
  measures "d92_3" distance of L9.end L10.end
  measures "d93_3" vertical distance of L10.end P0
  measures "d94_3" angle of L7 L10
extrude "Extrude1''''''''''" add sketch "Sketch2 (10)" along normal blind 24.5 separate body contours L8 L9 L10 L11 makes body 14 in component "Sensor-Holder East"
sketch "Sketch3 (7)" plane through (111.183, 111.183, 0) normal (0.707107, 0.707107, 0) x (0, 0, -1) in component "Sensor-Holder East"
  line L0 (60, 20.6824) -> (60, 45.6824)
  line L1 (60, 45.6824) -> (35.5, 45.6824)
  line L2 (35.5, 45.6824) -> (35.5, 20.6824)
  line L3 (35.5, 20.6824) -> (60, 20.6824)
  line L4 (60, 45.6824) -> (59, 45.6824)
  line L5 (59, 45.6824) -> (59, 20.6824)
  line L6 (59, 20.6824) -> (60, 20.6824)
  line L7 (60, 20.6824) -> (60, 45.6824)
  point P0 (60, 45.9619)
  dimension "d97_3" = 1
  constraint horizontal L4
  constraint vertical L5
  constraint horizontal L6
  constraint vertical L7
  constraint coincident L3 L5.end
  constraint coincident L0.end L1.start
  measures "d97_3" horizontal distance of L4.end P0
extrude "Extrude2'''''''''" add sketch "Sketch3 (7)" along normal blind 2 contours L0 L1 L3 L4 L5 L6 L7 bodies 14 in component "Sensor-Holder East"
sketch "Sketch4 (4)" plane through (111.183, 111.183, 0) normal (0.707107, 0.707107, 0) x (0, 0, -1) in component "Sensor-Holder East"
  line L0 (59, 20.6824) -> (59, 45.6824)
  line L1 (59, 45.6824) -> (35.5, 45.6824)
  line L2 (35.5, 45.6824) -> (35.5, 20.6824)
  line L3 (35.5, 20.6824) -> (59, 20.6824)
  circle A0 centre (38.5, 38.6824) radius 1.5
  circle A1 centre (38.5, 24.6824) radius 1.5
  dimension "d100_3" = 3
  dimension "d101_3" = 3
  dimension "d102_3" = 14
  dimension "d103_3" = 20.5
  dimension "d104_3" = 7
  dimension "d105_3" = 20.5
  measures "d100_3" diameter of A0
  measures "d101_3" diameter of A1
  measures "d102_3" distance of A0.centre A1.centre
  measures "d103_3" horizontal distance of L0.end A0.centre
  measures "d104_3" vertical distance of L1.end A0.centre
  measures "d105_3" horizontal distance of L0.start A1.centre
extrude "Extrude3'''''''" add sketch "Sketch4 (4)" along normal blind 3 contours A0 bodies 14 in component "Sensor-Holder East"
extrude "Extrude4''''''" add sketch "Sketch4 (4)" along normal up to surface (3 mm away) contours A1 bodies 14 in component "Sensor-Holder East"
sketch "Sketch1 (10)" plane through (111.183, 111.183, 0) normal (0.707107, 0.707107, 0) x (0, 0, -1) in component "Sensor West (1)"
  circle A0 centre (38.5, 24.6824) radius 1.5
  circle A1 centre (38.5, 38.6824) radius 1.5
  line L0 (59, 20.6824) -> (59, 45.6824)
  line L1 (59, 45.6824) -> (35.5, 45.6824)
  line L2 (35.5, 45.6824) -> (35.5, 20.6824)
  line L3 (35.5, 20.6824) -> (59, 20.6824)
  line L4 (59, 53.6824) -> (36, 53.6824)
  line L5 (36, 53.6824) -> (36, 7.6824)
  line L6 (36, 7.6824) -> (59, 7.6824)
  line L7 (59, 7.6824) -> (59, 53.6824)
  line L8 (60, 35.3553) -> (60, 247.4874)
  dimension "d111_3" = 8
  dimension "d113_3" = 46
  dimension "d114_3" = 23
  dimension "d115_3" = 1
  constraint horizontal L4
  constraint vertical L5
  constraint horizontal L6
  constraint vertical L7
  measures "d111_3" vertical distance of L1.end L4.end
  measures "d113_3" distance of L4.end L5.end
  measures "d114_3" distance of L5.end L6.end
  measures "d115_3" distance of L4.start L8
extrude "Extrude1'''''''''''" add sketch "Sketch1 (10)" along normal blind 1.6 separate body contours L0 L1 L3 L5 L7 | L3 L5 L6 L7 | L1 L4 L5 L7 makes body 15 in component "Sensor West (1)"
sketch "Sketch2 (11)" plane through (112.3143, 112.3143, 0) normal (0.707107, 0.707107, 0) x (0, 0, -1) in component "Sensor West (1)"
  circle A0 centre (38.5, 24.6824) radius 1.5
  circle A1 centre (38.5, 38.6824) radius 1.5
  line L0 (59, 7.6824) -> (59, 53.6824)
  line L1 (59, 53.6824) -> (36, 53.6824)
  line L2 (36, 53.6824) -> (36, 7.6824)
  line L3 (36, 7.6824) -> (59, 7.6824)
  circle A2 centre (44, 46.6824) radius 3
  line L4 (37.0281, 7.6824) -> (56, 7.6824)
  line L5 (36, 7.6824) -> (59, 7.6824)
  line L6 (59, 7.6824) -> (59, 16.3824)
  line L7 (59, 16.3824) -> (36, 16.3824)
  line L8 (36, 16.3824) -> (36, 7.6824)
  line L9 (44, 46.6824) -> (59, 46.6824)
  dimension "d119_3" = 7
  dimension "d124_3" = 6
  dimension "d125_3" = 8
  dimension "d126_3" = 8.7
  constraint horizontal L4
  constraint coincident L3 L4.start
  constraint horizontal L5
  constraint vertical L6
  constraint horizontal L7
  constraint vertical L8
  constraint coincident L0 L6.end
  constraint coincident L2.end L3.start
  constraint coincident A2.centre L9.start
  constraint coincident L0 L9.end
  constraint perpendicular L0 L9
  measures "d119_3" vertical distance of L1.end A2.centre
  measures "d124_3" diameter of A2
  measures "d125_3" horizontal distance of L1.end A2.centre
  measures "d126_3" distance of L2.end L7.end
extrude "Extrude2''''''''''" add sketch "Sketch2 (11)" along normal blind 3 contours A2 bodies 15 in component "Sensor West (1)"
extrude "Extrude4'''''''" add sketch "Sketch2 (11)" along normal blind 8.9 contours L0 L2 L3 L4 L5 L6 L7 L8 bodies 15 in component "Sensor West (1)"
sketch "Sketch2 (12)" plane through (0, 0, -59) normal (0, 0, 1) x (1, 0, 0) in component "Help lines"
  circle A0 centre (160, 225) radius 115
  circle A1 centre (160, 225) radius 118
  line L0 (160, 225) -> (85, 150)
  line L1 (85, 150) -> (76.5614, 141.5614)
  line L2 (160, 225) -> (235, 150)
  line L3 (235, 150) -> (243.4386, 141.5614)
  line L4 (160, 225) -> (85, 300)
  line L5 (85, 300) -> (76.5614, 308.4386)
  line L6 (160, 225) -> (235, 300)
  line L7 (235, 300) -> (243.4386, 308.4386)
  constraint coincident A0.centre A1.centre
  constraint coincident A1 L1.end
  constraint parallel L0 L1
  constraint perpendicular L0 L2
  constraint coincident A1 L3.end
  constraint parallel L2 L3
  constraint parallel L2 L4
  constraint coincident A1 L5.end
  constraint parallel L4 L5
  constraint perpendicular L4 L6
  constraint coincident A1 L7.end
  constraint parallel L6 L7
sketch "Sketch1 (11)" plane through (0, 0, -35.4282) normal (0, 0, 1) x (1, 0, 0) in component "Target holder bottom"
  line L0 (85.3026, 113.6358) -> (93.7879, 122.121)
  line L1 (61.9731, 140.0758) -> (257.9731, 140.0758)
  line L2 (257.9731, 140.0758) -> (257.9731, 125.0758)
  line L3 (257.9731, 125.0758) -> (61.9731, 125.0758)
  line L4 (61.9731, 125.0758) -> (61.9731, 140.0758)
  line L5 (271.4131, 150.4053) -> (262.9278, 158.8906)
  line L6 (262.9278, 158.8906) -> (245.2502, 141.2129)
  line L7 (257.9731, 136.9653) -> (271.4131, 150.4053)
  line L8 (262.9278, 158.8906) -> (245.2502, 141.2129)
  line L9 (246.3873, 140.0758) -> (245.2502, 141.2129)
  line L10 (271.4131, 150.4053) -> (262.9278, 158.8906)
  line L11 (271.4131, 150.4053) -> (257.9731, 136.9653)
  line L12 (73.8626, 125.0758) -> (85.3026, 113.6358)
  line L13 (93.7879, 122.121) -> (85.3026, 113.6358)
  line L14 (93.7879, 122.121) -> (90.8331, 125.0758)
  line L15 (73.8626, 125.0758) -> (85.3026, 113.6358)
  line L16 (93.7879, 122.121) -> (90.8331, 125.0758)
  line L17 (246.3873, 140.0758) -> (245.2502, 141.2129)
  line L18 (262.9278, 158.8906) -> (271.4131, 150.4053)
  line L19 (264.342, 157.4764) -> (269.9989, 151.8195)
  line L20 (269.9989, 151.8195) -> (271.0596, 152.8802)
  line L21 (271.0596, 152.8802) -> (265.4027, 158.537)
  line L22 (265.4027, 158.537) -> (264.342, 157.4764)
  line L23 (268.5847, 147.5769) -> (256.5639, 135.5561)
  line L24 (256.5639, 135.5561) -> (257.6245, 134.4954)
  line L25 (257.6245, 134.4954) -> (269.6453, 146.5162)
  line L26 (269.6453, 146.5162) -> (268.5847, 147.5769)
  line L27 (246.3873, 140.0758) -> (252.3212, 134.1419)
  line L28 (252.3212, 134.1419) -> (251.2606, 133.0812)
  line L29 (251.2606, 133.0812) -> (245.3266, 139.0151)
  line L30 (245.3266, 139.0151) -> (246.3873, 140.0758)
  line L31 (82.4742, 116.4642) -> (70.4534, 128.485)
  line L32 (70.4534, 128.485) -> (69.3927, 127.4243)
  line L33 (69.3927, 127.4243) -> (81.4135, 115.4035)
  line L34 (81.4135, 115.4035) -> (82.4742, 116.4642)
  line L35 (86.7168, 115.05) -> (92.3737, 120.7068)
  line L36 (92.3737, 120.7068) -> (93.4343, 119.6462)
  line L37 (93.4343, 119.6462) -> (87.7775, 113.9893)
  line L38 (87.7775, 113.9893) -> (86.7168, 115.05)
  line L39 (67.6249, 131.3134) -> (85.3026, 113.6358)
  line L40 (76.1102, 139.7987) -> (67.6249, 131.3134)
  line L41 (69.0391, 132.7276) -> (74.696, 138.3845)
  line L42 (74.696, 138.3845) -> (73.6353, 139.4452)
  line L43 (73.6353, 139.4452) -> (67.9785, 133.7883)
  line L44 (67.9785, 133.7883) -> (69.0391, 132.7276)
  point P0 (84.9731, 150.0758)
  point P1 (253.7354, 132.7276)
  dimension "d136" = 10
  dimension "d137" = 23
  dimension "d138" = 15
  dimension "d139" = 196
  dimension "d144" = 2
  dimension "d145" = 2
  dimension "d146" = 1.5
  dimension "d147" = 4
  dimension "d148" = 4
  dimension "d149" = 1.5
  dimension "d150" = 1.5
  dimension "d151" = 2
  dimension "d156" = 1.5
  dimension "d158" = 1.5
  dimension "d159" = 1.5
  dimension "d160" = 2
  dimension "d161" = 2
  dimension "d162" = 2
  dimension "d163" = 2
  dimension "d164" = 4
  dimension "d166" = 4
  constraint horizontal L1
  constraint vertical L2
  constraint horizontal L3
  constraint vertical L4
  constraint coincident L2 L7.start
  constraint coincident L5.start L7.end
  constraint coincident L5.end L6.start
  constraint coincident L6.end L8.end
  constraint coincident L1 L9.start
  constraint perpendicular L5 L11
  constraint coincident L3 L12.start
  constraint coincident L0.start L12.end
  constraint coincident L0.end L13.start
  constraint coincident L3 L14.end
  constraint perpendicular L0 L15
  constraint perpendicular L13 L16
  constraint perpendicular L8 L17
  constraint perpendicular L19 L20
  constraint parallel L19 L21
  constraint parallel L20 L22
  constraint coincident L5 L19.end
  constraint parallel L5 L19
  constraint perpendicular L23 L24
  constraint parallel L23 L25
  constraint parallel L24 L26
  constraint coincident L11 L23.end
  constraint perpendicular L21 L23
  constraint perpendicular L27 L28
  constraint parallel L27 L29
  constraint parallel L28 L30
  constraint parallel L9 L27
  constraint perpendicular L31 L32
  constraint parallel L31 L33
  constraint parallel L32 L34
  constraint parallel L12 L31
  constraint coincident L12 L31.start
  constraint perpendicular L35 L36
  constraint parallel L35 L37
  constraint parallel L36 L38
  constraint coincident L0 L35.end
  constraint perpendicular L12 L35
  constraint perpendicular L41 L42
  constraint parallel L41 L43
  constraint parallel L42 L44
  constraint coincident L40 L41.end
  constraint coincident L40 L41.start
  measures "d136" vertical distance of L1.start P0
  measures "d137" horizontal distance of L1.start P0
  measures "d138" distance of L1.start L3.end
  measures "d139" distance of L2.end L3.end
  measures "d144" distance of L5.start L19.end
  measures "d145" distance of L5.end L19.start
  measures "d146" distance of L19.end L20.end
  measures "d147" distance of L5.start L23.start
  measures "d148" distance of L23.end P1
  measures "d149" distance of L23.start L25.end
  measures "d150" distance of L9.start L29.end
  measures "d151" distance of L27.end P1
  measures "d156" distance of L35.start L37.end
  measures "d158" distance of L31.start L33.end
  measures "d159" distance of L41.start L43.end
  measures "d160" distance of L39.start L41.start
  measures "d161" distance of L40.start L41.end
  measures "d162" distance of L0.end L35.end
  measures "d163" distance of L0.start L35.start
  measures "d164" distance of L0.start L31.start
  measures "d166" distance of L31.end L39.start
extrude "Extrude1''''''''''''" add sketch "Sketch1 (11)" along normal blind 10 separate body contours L27 L28 L29 L30 | L1 L2 L3 L4 L23 L24 L25 L31 L32 L33 L39 | L3 L31 L32 L33 L39 | L2 L23 L24 L25 | L40 L41 L42 L43 L44 makes body 16 in component "Target holder bottom"
sketch "Sketch1 (12)" plane through (0, 0, -35.4282) normal (0, 0, 1) x (1, 0, 0) in component "Target holder right"
  line L0 (253.7354, 132.7276) -> (271.4131, 150.4053)
  line L1 (271.4131, 150.4053) -> (262.9278, 158.8906)
  line L2 (262.9278, 158.8906) -> (245.2501, 141.2129)
  line L3 (245.2501, 141.2129) -> (253.7354, 132.7276)
  line L4 (243, 140) -> (258, 140)
  line L5 (258, 140) -> (258, 310)
  line L6 (258, 310) -> (243, 310)
  line L7 (243, 310) -> (243, 140)
  line L8 (258, 140) -> (243, 140)
  line L9 (243, 140) -> (243, 310)
  line L10 (243, 310) -> (258, 310)
  line L11 (258, 310) -> (258, 140)
  constraint horizontal L8
  constraint vertical L9
  constraint horizontal L10
  constraint vertical L11
  constraint coincident L6.end L7.start
  constraint coincident L4.end L5.start
extrude "Extrude1'''''''''''''" add sketch "Sketch1 (12)" along normal blind 10 separate body contours L2 L3 L4 L5 L6 L7 L8 L9 L10 L11 | L2 L3 L4 L5 L8 L11 makes body 17 in component "Target holder right"
sketch "Sketch1 (13)" plane through (0, 0, -35.4282) normal (0, 0, 1) x (1, 0, 0) in component "Target holder left"
  line L0 (67.6249, 131.3134) -> (85.3026, 113.6358)
  line L1 (85.3026, 113.6358) -> (93.7879, 122.121)
  line L2 (93.7879, 122.121) -> (76.1102, 139.7987)
  line L3 (76.1102, 139.7987) -> (67.6249, 131.3134)
  line L4 (77, 140) -> (77, 310)
  line L5 (77, 310) -> (62, 310)
  line L6 (62, 310) -> (62, 140)
  line L7 (62, 140) -> (77, 140)
  line L8 (77, 140) -> (62, 140)
  line L9 (62, 140) -> (62, 310)
  line L10 (62, 310) -> (77, 310)
  line L11 (77, 310) -> (77, 140)
  constraint horizontal L8
  constraint vertical L9
  constraint horizontal L10
  constraint vertical L11
  constraint coincident L5.end L6.start
  constraint coincident L4.start L7.end
extrude "Extrude1''''''''''''''" add sketch "Sketch1 (13)" along normal blind 10 separate body contours L4 L5 L6 L7 L8 L9 L10 L11 makes body 7 in component "Target holder left"
sketch "Sketch2 (13)" plane through (77, 0, 0) normal (1, 0, 0) x (0, 0, -1) in component "Target holder left"
  line L0 (35.4282, 140) -> (35.4282, 310)
  line L1 (35.4282, 310) -> (25.4282, 310)
  line L2 (25.4282, 310) -> (25.4282, 140)
  line L3 (25.4282, 140) -> (35.4282, 140)
  line L4 (34.8282, 140) -> (33.3282, 140)
  line L5 (33.3282, 140) -> (33.3282, 310)
  line L6 (33.3282, 310) -> (34.8282, 310)
  line L7 (34.8282, 310) -> (34.8282, 140)
  dimension "d171" = 1.5
  dimension "d172" = 0.6
  constraint horizontal L4
  constraint vertical L5
  constraint horizontal L6
  constraint vertical L7
  constraint coincident L1 L5.end
  constraint coincident L3 L4.start
  measures "d171" distance of L5.end L6.end
  measures "d172" distance of L0.end L6.end
extrude "Extrude5" cut sketch "Sketch2 (13)" against normal blind 3 contours L1 L3 L4 L5 L6 L7 bodies 16 in component "Target holder bottom"
extrude "Extrude2'''''''''''" cut sketch "Sketch2 (13)" against normal blind 3 contours L1 L3 L4 L5 L6 L7 bodies 7 in component "Target holder left"
sketch "Sketch2 (14)" plane through (243, 0, 0) normal (-1, 0, 0) x (0, 0, 1) in component "Target holder right"
  line L0 (-35.4282, 310) -> (-35.4282, 140)
  line L1 (-35.4282, 140) -> (-25.4282, 140)
  line L2 (-25.4282, 140) -> (-25.4282, 310)
  line L3 (-25.4282, 310) -> (-35.4282, 310)
  line L4 (-33.3282, 310) -> (-34.8282, 310)
  line L5 (-34.8282, 310) -> (-34.8282, 140)
  line L6 (-34.8282, 140) -> (-33.3282, 140)
  line L7 (-33.3282, 140) -> (-33.3282, 310)
  dimension "d177" = 1.5
  dimension "d178" = 0.6
  constraint horizontal L4
  constraint vertical L5
  constraint horizontal L6
  constraint vertical L7
  constraint coincident L1 L5.end
  constraint coincident L3 L4.start
  measures "d177" distance of L5.end L6.end
  measures "d178" distance of L0.end L5.end
extrude "Extrude6" cut sketch "Sketch2 (14)" against normal blind 3 contours L1 L3 L4 L5 L6 L7 bodies 16 in component "Target holder bottom"
extrude "Extrude2''''''''''''" cut sketch "Sketch2 (14)" against normal blind 3 contours L1 L3 L4 L5 L6 L7 bodies 17 in component "Target holder right"
sketch "Sketch2 (15)" plane through (0, 140.0758, 0) normal (0, 1, 0) x (-1, 0, 0) in component "Target holder bottom"
  line L0 (-246, -33.3282) -> (-243, -33.3282)
  line L1 (-243, -33.3282) -> (-243, -34.8282)
  line L2 (-243, -34.8282) -> (-246, -34.8282)
  line L3 (-246, -34.8282) -> (-246, -33.3282)
  line L4 (-74, -34.8282) -> (-77, -34.8282)
  line L5 (-77, -34.8282) -> (-77, -33.3282)
  line L6 (-77, -33.3282) -> (-74, -33.3282)
  line L7 (-74, -33.3282) -> (-74, -34.8282)
  line L8 (-257.9731, -35.4282) -> (-61.9731, -35.4282)
  line L9 (-61.9731, -35.4282) -> (-61.9731, -25.4282)
  line L10 (-61.9731, -25.4282) -> (-257.9731, -25.4282)
  line L11 (-257.9731, -25.4282) -> (-257.9731, -35.4282)
  line L12 (-66.9731, -32.4282) -> (-72.9731, -32.4282)
  line L13 (-72.9731, -32.4282) -> (-72.9731, -28.4282)
  line L14 (-72.9731, -28.4282) -> (-66.9731, -28.4282)
  line L15 (-66.9731, -28.4282) -> (-66.9731, -32.4282)
  line L16 (-246.9731, -32.4282) -> (-252.9731, -32.4282)
  line L17 (-252.9731, -32.4282) -> (-252.9731, -28.4282)
  line L18 (-252.9731, -28.4282) -> (-246.9731, -28.4282)
  line L19 (-246.9731, -28.4282) -> (-246.9731, -32.4282)
  dimension "d183" = 3
  dimension "d184" = 3
  dimension "d185" = 5
  dimension "d186" = 6
  dimension "d187" = 6
  dimension "d188" = 5
  dimension "d189" = 3
  dimension "d190" = 3
  constraint horizontal L12
  constraint vertical L13
  constraint horizontal L14
  constraint vertical L15
  constraint horizontal L16
  constraint vertical L17
  constraint horizontal L18
  constraint vertical L19
  measures "d183" vertical distance of L9.end L14.end
  measures "d184" vertical distance of L8.end L12.start
  measures "d185" horizontal distance of L9.end L14.end
  measures "d186" distance of L13.end L14.end
  measures "d187" distance of L17.end L18.end
  measures "d188" horizontal distance of L10.end L17.end
  measures "d189" vertical distance of L10.end L17.end
  measures "d190" vertical distance of L8.start L16.end
extrude "Extrude7" add sketch "Sketch2 (15)" along normal blind 5 contours L12 L13 L14 L15 | L16 L17 L18 L19 bodies 16 in component "Target holder bottom"